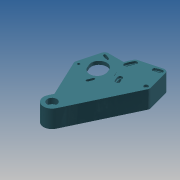
# Autodesk Inventor part: top plate
Saved by Autodesk Inventor 2013 (Build 170138000, 138)
## iProperties
Created: 2017-03-31
Part Number: top plate
Material: Generic
Document SubType Name: Modeling
Designer: employee
Density: 1 g/cm^3
Author: employee
Autodesk Inventor part; units mm, degrees
ref_plane "YZ Plane" through (0, 0, 0) normal (1, 0, 0) x (0, 1, 0)
ref_plane "XZ Plane" through (0, 0, 0) normal (0, 1, 0) x (-1, 0, 0)
ref_plane "XY Plane" through (0, 0, 0) normal (0, 0, 1) x (1, 0, 0)
sketch "Sketch1" plane through (0, 0, 0) normal (0, 0, 1) x (1, 0, 0)
  circle A0 centre (0, 0) radius 99 construction
  line L0 (0, 103.3586) -> (36.9795, 123.2713) construction
  line L1 (36.9795, 123.2713) -> (56.8922, 86.2918) construction
  line L2 (56.8922, 86.2918) -> (19.9127, 66.3791) construction
  line L3 (19.9127, 66.3791) -> (0, 103.3586) construction
  line L4 (19.9127, 66.3791) -> (0, 0) construction
  line L5 (34.7446, 115.8211) -> (7.4502, 101.1237) construction
  line L6 (7.4502, 101.1237) -> (22.1476, 73.8293) construction
  line L7 (22.1476, 73.8293) -> (49.442, 88.5267) construction
  line L8 (49.442, 88.5267) -> (34.7446, 115.8211) construction
  line L9 (45.2305, 125.1977) -> (56.1863, 84.6519) construction
  line L10 (56.1863, 84.6519) -> (15.6404, 73.696) construction
  line L11 (15.6404, 73.696) -> (4.6846, 114.2419) construction
  line L12 (30.4355, 99.4469) -> (28.9722, 94.6658) construction
  line L13 (0, 103.3586) -> (6.6568, 106.9431)
  line L14 (6.6568, 106.9431) -> (4.6846, 114.2419)
  line L15 (4.6846, 114.2419) -> (45.2305, 125.1977)
  line L16 (45.2305, 125.1977) -> (55.8891, 85.7517)
  line L17 (55.8891, 85.7517) -> (19.9127, 66.3791)
  line L18 (19.9127, 66.3791) -> (0, 103.3586)
  circle A1 centre (49.442, 88.5267) radius 1.75
  circle A2 centre (22.1476, 73.8293) radius 1.75
  circle A3 centre (7.4502, 101.1237) radius 1.75
  circle A4 centre (34.7446, 115.8211) radius 1.75
  line L19 (11.4289, 110.367) -> (41.3556, 118.4535) construction
  line L20 (41.3556, 118.4535) -> (49.442, 88.5267) construction
  line L21 (49.442, 88.5267) -> (19.5153, 80.4403) construction
  line L22 (19.5153, 80.4403) -> (11.4289, 110.367) construction
  circle A5 centre (19.5153, 80.4403) radius 1.75
  circle A6 centre (11.4289, 110.367) radius 1.75
  circle A7 centre (41.3556, 118.4535) radius 1.75
  point P0 (28.4461, 94.8252)
  point P1 (30.4355, 99.4469)
  dimension "d0" = 198
  dimension "d2" = 42
  dimension "d3" = 31
  dimension "d4" = 5.5
  dimension "d5" = 5.5
  dimension "d6" = 5
  dimension "d7" = 3.5
  dimension "d8" = 5.5
  dimension "d9" = 5.5
  constraints: 46 end point, 8 centre point, 8 coincident, 6 equal radius, 6 point on line, 3 collinear, 2 equal length, 2 point on circle, 1 parallel, 1 perpendicular, 1 vertical alignment, 28 other
  measures "d0" diameter of A0
  measures "d2" distance between parallel lines of L1 L3
  measures "d3" distance between parallel lines of L6 L8
  measures "d4" distance from line of L10 L7.end
  measures "d5" distance from line of L9 L7.end
  measures "d6" distance of L12.start L12.end
  measures "d7" diameter of A3
  measures "d8" distance between parallel lines of L22 L11
  measures "d9" distance between parallel lines of L21 L10
extrude "Extrusion1" add sketch "Sketch1" along normal blind 5
fillet "Fillet1" radius 5.5 5 edges at (4.6846, 114.2419, 2.5) (0, 103.3586, 2.5) (45.2305, 125.1977, 2.5) (19.9127, 66.3791, 2.5) (55.8891, 85.7517, 2.5)
sketch "Sketch2" plane through (0, 0, 5) normal (0, 0, 1) x (1, 0, 0)
  circle A0 centre (41.3556, 118.4535) radius 1.75 projected
  circle A1 centre (11.4289, 110.367) radius 1.75 projected
  circle A2 centre (19.5153, 80.4403) radius 1.75 projected
  circle A3 centre (34.7446, 115.8211) radius 1.75 projected
  circle A4 centre (7.4502, 101.1237) radius 1.75 projected
  circle A5 centre (22.1476, 73.8293) radius 1.75 projected
  circle A6 centre (49.442, 88.5267) radius 1.75 projected
  arc A7 (12.9463, 109.4952) -> (9.1264, 100.6208) centre (49.442, 88.5267) ccw
  arc A8 (9.9115, 111.2388) -> (5.774, 101.6265) centre (49.442, 88.5267) ccw
  arc A9 (41.8121, 116.7641) -> (35.5743, 114.2803) centre (49.442, 88.5267) ccw
  arc A10 (21.2047, 80.8968) -> (23.6885, 74.659) centre (49.442, 88.5267) ccw
  arc A11 (40.8991, 120.1429) -> (33.9149, 117.362) centre (49.442, 88.5267) ccw
  arc A12 (17.8259, 79.9838) -> (20.6068, 72.9996) centre (49.442, 88.5267) ccw
  point P0 (0, 0)
  constraints: 24 point on circle, 6 centre point, 6 tangent, 4 coincident
extrude "Extrusion2" cut sketch "Sketch2" against normal through all contours A0 A9 A3 A11 | A1 A7 A4 A8 | A2 A10 A5 A12
sketch "Sketch3" plane through (0, 0, 5) normal (0, 0, 1) x (1, 0, 0)
  arc A0 (9.9942, 115.6766) -> (6.1193, 108.9323) centre (11.4289, 110.367) ccw projected
  line L0 (6.1193, 108.9323) -> (6.6568, 106.9431) projected
  line L1 (6.6568, 106.9431) -> (4.8426, 105.9662) projected
  arc A1 (4.8426, 105.9662) -> (2.6076, 98.516) centre (7.4502, 101.1237) ccw projected
  circle A2 centre (49.442, 88.5267) radius 1.75 projected
  arc A3 (6.6599, 113.107) -> (2.1821, 102.704) centre (49.442, 88.5267) ccw
  point P0 (0, 0)
  constraints: 4 point on circle, 1 centre point, 1 coincident, 1 tangent
extrude "Extrusion3" add sketch "Sketch3" against normal up to surface (5 mm away) contours A0 L0 L1 A1 A3
mirror "Mirror1" about plane through (0, 0, 0) normal (1, 0, 0) of "Extrusion1", "Fillet1", "Extrusion2", "Extrusion3"
sketch "Sketch4" plane through (-49.442, 88.5267, 5) normal (0, 0, 1) x (0.9185232, 0.3953672, 0)
  arc A0 (-4.3097, 3.417) -> (-4.3097, -3.417) centre (0, 0) ccw projected
  line L0 (14.9499, -27.7083) -> (-4.3097, -3.417) projected
  arc A1 (14.9499, -27.7083) -> (22.6767, -28.601) centre (19.2596, -24.2913) ccw projected
  line L1 (46.968, -9.3414) -> (22.6767, -28.601) projected
  arc A2 (46.968, -9.3414) -> (49.0146, -5.6629) centre (43.5509, -5.0316) ccw projected
  arc A3 (49.0146, -5.6629) -> (49.0146, 5.6629) centre (0, 0) ccw projected
  arc A4 (49.0146, 5.6629) -> (46.968, 9.3414) centre (43.5509, 5.0316) ccw projected
  line L2 (22.6767, 28.601) -> (46.968, 9.3414) projected
  arc A5 (22.6767, 28.601) -> (14.9499, 27.7083) centre (19.2596, 24.2913) ccw projected
  arc A6 (95.4804, -6.6778) -> (87.9658, -6.4708) centre (90.8273, -39.0955) ccw projected
  arc A7 (94.9832, -10.1423) -> (95.4804, -6.6778) centre (95.2318, -8.41) ccw projected
  arc A8 (94.9832, -10.1423) -> (88.2716, -9.9574) centre (90.8273, -39.0955) ccw projected
  arc A9 (87.9658, -6.4708) -> (88.2716, -9.9574) centre (88.1187, -8.2141) ccw projected
  arc A10 (61.8741, -34.9397) -> (61.6892, -41.6513) centre (90.8273, -39.0955) ccw projected
  arc A11 (58.2026, -41.9571) -> (61.6892, -41.6513) centre (59.9459, -41.8042) ccw projected
  arc A12 (58.4096, -34.4424) -> (58.2026, -41.9571) centre (90.8273, -39.0955) ccw projected
  arc A13 (61.8741, -34.9397) -> (58.4096, -34.4424) centre (60.1418, -34.6911) ccw projected
  arc A14 (63.4972, -2.6049) -> (55.8964, -9.7982) centre (90.8273, -39.0955) ccw projected
  arc A15 (65.5953, -5.4062) -> (63.4972, -2.6049) centre (64.5463, -4.0056) ccw projected
  arc A16 (65.5953, -5.4062) -> (58.5781, -12.0473) centre (90.8273, -39.0955) ccw projected
  arc A17 (55.8964, -9.7982) -> (58.5781, -12.0473) centre (57.2372, -10.9228) ccw projected
  arc A18 (91.3079, -44.5745) -> (96.2715, -39.877) centre (90.8273, -39.0955) ccw projected
  line L3 (96.2715, -39.877) -> (100.676, -9.1914) projected
  arc A19 (100.676, -9.1914) -> (96.0132, -2.9658) centre (95.2318, -8.41) ccw projected
  line L4 (96.0132, -2.9658) -> (65.3277, 1.4387) projected
  arc A20 (65.3277, 1.4387) -> (61.2492, 0.3966) centre (64.5463, -4.0056) ccw projected
  arc A21 (61.2492, 0.3966) -> (53.0232, -7.3884) centre (90.8273, -39.0955) ccw projected
  arc A22 (53.0232, -7.3884) -> (51.7583, -11.4033) centre (57.2372, -10.9228) ccw projected
  line L5 (51.7583, -11.4033) -> (54.4669, -42.2848) projected
  arc A23 (54.4669, -42.2848) -> (60.4265, -47.2832) centre (59.9459, -41.8042) ccw projected
  line L6 (60.4265, -47.2832) -> (91.3079, -44.5745) projected
  circle A24 centre (90.8273, -39.0955) radius 1.75 projected
  circle A25 centre (10.4131, -100.8616) radius 12.5
  line L7 (18.6936, -110.2255) -> (94.4708, -43.2156)
  line L8 (-2.0798, -101.2839) -> (-5.4969, -0.1858)
  line L9 (21.4342, 29.3432) -> (97.4063, -3.3581)
  arc A26 (100.676, -9.1914) -> (96.0132, -2.9658) centre (95.2318, -8.41) ccw projected
  line L10 (-0.2455, -94.3313) -> (53.0232, -7.3884)
  dimension "d17" = 25
  constraints: 8 end point, 7 point on circle, 7 tangent, 1 centre point, 1 coincident
  measures "d17" diameter of A25
extrude "Extrusion4" add sketch "Sketch4" against normal blind 5 contours A0 L0 A1 L1 A2 A3 A4 L2 A5 L9 A19 L4 A20 A21 A22 L10 A25 L8 | A25 | L10 A22 L5 A23 L6 A18 L7 A25
extrude "Extrusion5" add sketch "Sketch4" along normal blind 21 contours A25 | L10 A22 L5 A23 L6 A18 L7 A25 | L10 A21 A20 L4 A19 L3 A18 L6 A23 L5 A22
sketch "Sketch5" plane through (-49.442, 88.5267, 26) normal (0, 0, 1) x (0.9185232, 0.3953672, 0)
  arc A0 (-0.2455, -94.3313) -> (18.6936, -110.2255) centre (10.4131, -100.8616) ccw projected
  circle A1 centre (10.4131, -100.8616) radius 4.25
  dimension "d23" = 8.5
  constraints: 1 centre point, 1 coincident
  measures "d23" diameter of A1
extrude "Extrusion6" cut sketch "Sketch5" against normal through all
sketch "Sketch6" plane through (0, 0, 5) normal (0, 0, 1) x (1, 0, 0)
  arc A0 (-9.1264, 100.6208) -> (-5.774, 101.6265) centre (-7.4502, 101.1237) ccw projected
  arc A1 (-9.9115, 111.2388) -> (-12.9463, 109.4952) centre (-11.4289, 110.367) ccw projected
  arc A2 (-35.5743, 114.2803) -> (-41.8121, 116.7641) centre (-49.442, 88.5267) ccw projected
  line L0 (-11.4289, 110.367) -> (-49.442, 88.5267) construction
  line L1 (-7.4502, 101.1237) -> (-49.442, 88.5267) construction
  circle A3 centre (-30.4355, 99.4469) radius 11.25
  circle A4 centre (-28.4461, 94.8252) radius 11.25
  dimension "d28" = 22.5
  constraints: 4 end point, 2 centre point, 2 midpoint, 1 coincident, 1 equal radius
  measures "d28" diameter of A3
extrude "Extrusion7" cut sketch "Sketch6" against normal through all
sketch "Sketch7" plane through (0, 0, 5) normal (0, 0, 1) x (1, 0, 0)
  arc A0 (-19.3691, 101.4713) -> (-39.5125, 92.8008) centre (-30.4355, 99.4469) ccw projected
  arc A1 (-39.5125, 92.8008) -> (-19.3691, 101.4713) centre (-28.4461, 94.8252) ccw projected
  arc A2 (-35.5743, 114.2803) -> (-41.8121, 116.7641) centre (-49.442, 88.5267) ccw projected
  arc A3 (-39.2217, 91.5927) -> (-40.1901, 93.8424) centre (-49.442, 88.5267) ccw
  arc A4 (-17.6705, 98.0577) -> (-20.6808, 105.0514) centre (-49.442, 88.5267) ccw
  constraints: 8 point on circle, 2 centre point, 2 coincident, 2 tangent
extrude "Extrusion8" cut sketch "Sketch7" against normal through all contours A0 A4 A1 | A0 A1 A3
sketch "Sketch8" plane through (-49.442, 88.5267, 26) normal (0, 0, 1) x (0.9185232, 0.3953672, 0)
  arc A0 (65.5953, -5.4062) -> (63.4972, -2.6049) centre (64.5463, -4.0056) ccw projected
  arc A1 (65.5953, -5.4062) -> (58.5781, -12.0473) centre (90.8273, -39.0955) ccw projected
  arc A2 (55.8964, -9.7982) -> (58.5781, -12.0473) centre (57.2372, -10.9228) ccw projected
  arc A3 (63.4972, -2.6049) -> (55.8964, -9.7982) centre (90.8273, -39.0955) ccw projected
  arc A4 (58.2026, -41.9571) -> (61.6892, -41.6513) centre (59.9459, -41.8042) ccw projected
  arc A5 (58.4096, -34.4424) -> (58.2026, -41.9571) centre (90.8273, -39.0955) ccw projected
  arc A6 (61.8741, -34.9397) -> (58.4096, -34.4424) centre (60.1418, -34.6911) ccw projected
  arc A7 (61.8741, -34.9397) -> (61.6892, -41.6513) centre (90.8273, -39.0955) ccw projected
  arc A8 (94.9832, -10.1423) -> (95.4804, -6.6778) centre (95.2318, -8.41) ccw projected
  arc A9 (94.9832, -10.1423) -> (88.2716, -9.9574) centre (90.8273, -39.0955) ccw projected
  arc A10 (87.9658, -6.4708) -> (88.2716, -9.9574) centre (88.1187, -8.2141) ccw projected
  arc A11 (95.4804, -6.6778) -> (87.9658, -6.4708) centre (90.8273, -39.0955) ccw projected
  circle A12 centre (90.8273, -39.0955) radius 1.75 projected
  arc A13 (66.3447, -6.4067) -> (59.5358, -12.8506) centre (90.8273, -39.0955) ccw
  arc A14 (66.3447, -6.4067) -> (62.7479, -1.6044) centre (64.5463, -4.0056) ccw
  arc A15 (62.7479, -1.6044) -> (54.9387, -8.9949) centre (90.8273, -39.0955) ccw
  arc A16 (54.9387, -8.9949) -> (59.5358, -12.8506) centre (57.2372, -10.9228) ccw
  arc A17 (94.8056, -11.3796) -> (88.3808, -11.2026) centre (90.8273, -39.0955) ccw
  arc A18 (94.8056, -11.3796) -> (95.658, -5.4404) centre (95.2318, -8.41) ccw
  arc A19 (95.658, -5.4404) -> (87.8565, -5.2256) centre (90.8273, -39.0955) ccw
  arc A20 (87.8565, -5.2256) -> (88.3808, -11.2026) centre (88.1187, -8.2141) ccw
  circle A21 centre (90.8273, -39.0955) radius 3
  arc A22 (56.9574, -42.0663) -> (62.9344, -41.5421) centre (59.9459, -41.8042) ccw
  arc A23 (57.1723, -34.2648) -> (56.9574, -42.0663) centre (90.8273, -39.0955) ccw
  arc A24 (63.1114, -35.1173) -> (57.1723, -34.2648) centre (60.1418, -34.6911) ccw
  arc A25 (63.1114, -35.1173) -> (62.9344, -41.5421) centre (90.8273, -39.0955) ccw
  dimension "d34" = 6
  constraints: 24 point on circle, 13 centre point, 3 equal radius, 9 other
  measures "d34" diameter of A21
extrude "Extrusion9" cut sketch "Sketch8" against normal blind 3
sketch "Sketch9" plane through (-49.442, 88.5267, 26) normal (0, 0, 1) x (0.9185232, 0.3953672, 0)
  circle A0 centre (10.4131, -100.8616) radius 4.25 projected
  arc A1 (-0.2455, -94.3313) -> (18.6936, -110.2255) centre (10.4131, -100.8616) ccw projected
  circle A2 centre (10.4131, -100.8616) radius 7
  dimension "d38" = 14
  constraints: 1 centre point, 1 coincident
  measures "d38" diameter of A2
extrude "Extrusion10" cut sketch "Sketch9" against normal blind 8
sketch "Sketch20" plane through (-49.442, 88.5267, 26) normal (0, 0, 1) x (0.9185232, 0.3953672, 0)
  arc A0 (56.9574, -42.0663) -> (62.9344, -41.5421) centre (59.9459, -41.8042) ccw projected
  arc A1 (54.9387, -8.9949) -> (59.5358, -12.8506) centre (57.2372, -10.9228) ccw projected
  line L0 (53.0232, -7.3884) -> (-0.2455, -94.3313) projected
  line L1 (18.6936, -110.2255) -> (94.4708, -43.2156) projected
  arc A2 (2.1326, -91.4977) -> (-0.2455, -94.3313) centre (10.4131, -100.8616) ccw
  line L2 (2.1326, -91.4977) -> (54.7057, -45.0072)
  line L3 (57.2372, -10.9228) -> (59.9459, -41.8042) construction
  line L4 (54.7057, -45.0072) -> (51.6086, -9.6972)
  dimension "d57" = 25
  dimension "d58" = 5.5
  constraints: 6 end point, 2 parallel, 2 point on circle, 2 tangent, 1 centre point, 1 point on line
  measures "d57" distance between parallel lines of L2 L1
  measures "d58" distance between parallel lines of L3 L4
extrude "Extrusion11" cut sketch "Sketch20" against normal up to surface (21 mm away)
fillet "Fillet4" radius 5.5 2 edges at (1.7956, 100.024, 15.5) (18.6008, 68.8155, 15.5)
body "Solid1"
